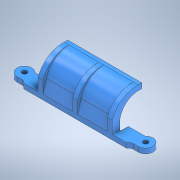
# Autodesk Inventor part: Battery mount front
Saved by Autodesk Inventor 2022 (Build 260153000, 153)
## iProperties
Created: 2023-01-31
Part Number: Battery mount front
Material: Generic
Document SubType Name: Modeling
Designer: scott
Density: 1 g/cm^3
Appearance: Default
Author: scott
Autodesk Inventor part; units mm, degrees
ref_plane "YZ Plane" through (0, 0, 0) normal (1, 0, 0) x (0, 1, 0)
ref_plane "XZ Plane" through (0, 0, 0) normal (0, 1, 0) x (-1, 0, 0)
sketch "Sketch1" plane through (0, 0, 0) normal (0, 1, 0) x (-1, 0, 0)
  line L0 (24.5, 6) -> (0, 6)
  line L1 (0, 6) -> (0, 0)
  line L2 (0, 0) -> (24.5, 0)
  line L3 (24.5, 0) -> (24.5, 6)
  circle A0 centre (24.5, 3) radius 3
  circle A1 centre (24.5, 3) radius 1
  line L4 (22.2639, 1) -> (0, 1)
  line L5 (0, 1) -> (0, 0)
  line L6 (0, 0) -> (22.2639, 0)
  line L7 (22.2639, 0) -> (22.2639, 1)
  line L8 (0, 4) -> (15.5, 4)
  line L9 (15.5, 4) -> (15.5, 1)
  line L10 (15.5, 1) -> (0, 1)
  line L11 (0, 1) -> (0, 4)
  line L12 (24.5, 3) -> (0, 3)
  line L13 (0, 3) -> (0, 7)
  line L14 (0, 7) -> (24.5, 7)
  line L15 (24.5, 7) -> (24.5, 3)
  line L16 (24.5, 7) -> (20.5, 7)
  line L17 (20.5, 7) -> (20.5, 6)
  line L18 (20.5, 6) -> (24.5, 6)
  line L19 (24.5, 6) -> (24.5, 7)
  circle A2 centre (22.5, 8) radius 2
  line L20 (15.5, 4) -> (15.5, 7)
  point P0 (22.5, 6)
  point P1 (20.7679, 7)
  point P2 (0, 6)
  point P3 (15.5, 3)
  point P4 (0, 3)
  point P5 (15.5, 6)
  point P6 (0, 6)
  dimension "d0" = 24.5
  dimension "d1" = 6
  dimension "d2" = 2
  dimension "d3" = 0
  dimension "d4" = 0
  dimension "d6" = 3
  dimension "d7" = 4
  dimension "d8" = 4
  dimension "d9" = 4
  dimension "d10" = 2
  dimension "d13" = 2
  dimension "d14" = 9
  constraints: 42 end point, 10 parallel, 6 perpendicular, 5 horizontal, 4 point on line, 3 centre point, 2 point on circle, 1 coincident, 1 midpoint, 1 tangent
  measures "d0" distance between parallel lines of L1 L3
  measures "d1" distance of L0.end L1.end
  measures "d2" diameter of A1
  measures "d3" distance from line of point (0, 0) L1
  measures "d4" distance from line of point (0, 0) L2
  measures "d6" distance of L8.end L9.end
  measures "d7" distance of L12.end L13.end
  measures "d8" distance from line of L17 A0.centre
  measures "d9" diameter of A2
  measures "d10" distance from line of L17 A2.centre
  measures "d13" distance from line of L4 A0.centre
  measures "d14" distance from line of L9 A0.centre
extrude "Extrusion1" add sketch "Sketch1" along normal blind 2 contours A0 L12 L9 L20 L0 | A0 L3 A1 | L3 A1 L12 A0 | L0 L17 L14 A2 | L12 A1 L3 A0 | A0 L4 L9 L12 | L0 L20 L14 L17 | L20 L8 L1 L0 | L0 L13 L14 L20
sketch "Sketch2" plane through (0, 0, 7) normal (1, 0, 0) x (0, 0, -1)
  line L0 (0, 2) -> (3, 2) projected
  line L1 (3, 2) -> (0, 2)
  line L2 (0, 2) -> (0, 12)
  line L3 (0, 12) -> (3, 12)
  line L4 (3, 12) -> (3, 2)
  line L5 (0, 12) -> (12, 12)
  line L6 (12, 12) -> (12, 9)
  line L7 (12, 9) -> (0, 9)
  line L8 (0, 9) -> (0, 12)
  line L9 (0, 0) -> (3, 0) projected
  circle A0 centre (10.5, 4.5) radius 7.5
  line L10 (3, 2) -> (6, 2) projected
  line L11 (0, 12) -> (12, 12)
  line L12 (12, 12) -> (12, 14)
  line L13 (12, 14) -> (0, 14)
  line L14 (0, 14) -> (0, 12)
  circle A1 centre (10.5, 4.5) radius 9.5
  line L15 (0, 2) -> (1.3214, 6.9501)
  point P0 (7, 0)
  point P1 (10.5, 14)
  point P2 (3, 4.5)
  point P3 (10.5, 12)
  dimension "d15" = 10
  dimension "d16" = 12
  dimension "d17" = 3
  dimension "d20" = 15
  dimension "d21" = 2.5
  dimension "d22" = 7.5
  dimension "d23" = 12
  dimension "d24" = 2
  constraints: 26 end point, 6 parallel, 4 horizontal, 3 perpendicular, 1 centre point, 1 coincident, 4 other
  measures "d15" distance of L1.end L2.end
  measures "d16" distance of L6.end L7.end
  measures "d17" distance of L5.end L6.end
  measures "d20" diameter of A0
  measures "d21" distance from line of L10 A0.centre
  measures "d22" distance from line of L4 A0.centre
  measures "d23" distance of L13.end L12.end
  measures "d24" distance of L12.end L11.end
extrude "Extrusion2" add sketch "Sketch2" against normal blind 15 contours L15 A1 L0 | A1 L7 L4 L0 | A1 L4 L7 | L4 L7 A0 | L4 A1 L5 A0 L7 | A1 L13 L12 | L12 L5 A1
mirror "Mirror1" about plane through (0, 0, 7) normal (1, 0, 0) of "Extrusion1", "Extrusion2"
ref_plane "Work Plane1" through (0, 2, 4) normal (1, 0, 0) x (0, 0, -1)
sketch "Sketch4" plane through (0, 2, 4) normal (1, 0, 0) x (0, 0, -1)
  line L0 (-3, 0) -> (-1.6786, 4.9501) projected
  line L1 (-3, 0) -> (-3, 4.9501)
  line L2 (-3, 4.9501) -> (-1.6786, 4.9501)
  arc A0 (7.5, 12) -> (-1.6786, 4.9501) centre (7.5, 2.5) ccw projected
  arc A1 (7.5, 12) -> (-3, 4.9501) centre (7.0292, 1.357) ccw
  circle A2 centre (7.5, 2.5) radius 9.5
  point P0 (4, -2)
  constraints: 4 end point, 2 centre point, 2 point on circle, 1 coincident, 1 concentric, 1 perpendicular, 1 vertical
extrude "Extrusion3" add sketch "Sketch4" along normal mid plane 2 contours L1 L2 L0 | L2 A1 A0
pattern_linear "Rectangular Pattern1" count 2 spacing 14 along (-1, 0, 0) count 2 spacing 14 along (1, 0, 0) of "Extrusion3"
sketch "Sketch5" plane through (-15, 0, 7) normal (-1, 0, 0) x (0, 0, 1)
  point P0 (-7, 0)
equation "\"d11\" = d2"
body "Solid1"
